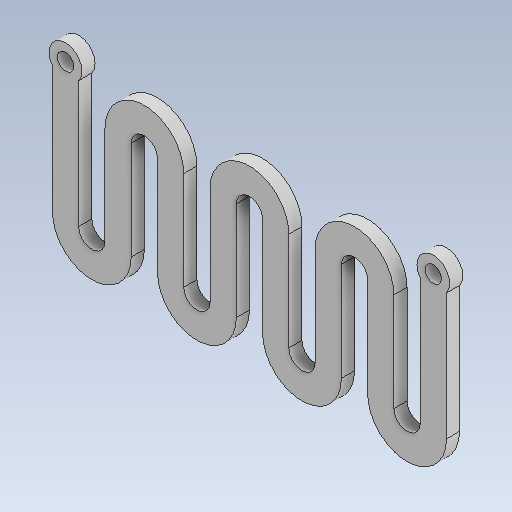
# Autodesk Inventor part: sensor2
Saved by Autodesk Inventor 2025.2 (Build 292293000, 293)
## iProperties
Created: 2025-01-23
Part Number: sensor2
Material: Genérico
Document SubType Name: Modeling
Designer: Gustavo Sousa
Density: 1 g/cm^3
Appearance: Padrão
Author: Gustavo Sousa
Autodesk Inventor part; units mm, degrees
ref_plane "YZ Plane" through (0, 0, 0) normal (1, 0, 0) x (0, 1, 0)
ref_plane "XZ Plane" through (0, 0, 0) normal (0, 1, 0) x (-1, 0, 0)
ref_plane "XY Plane" through (0, 0, 0) normal (0, 0, 1) x (1, 0, 0)
sketch "Esboço1" plane through (0, 0, 0) normal (0, 0, 1) x (1, 0, 0)
  arc A0 (-2600, 1100) -> (-3000, 1100) centre (-2800, 1250) ccw
  line L0 (-2800, 1250) -> (-2800, -825) construction
  line L1 (-3000, -825) -> (-3000, 1100)
  line L2 (-2600, -825) -> (-2600, 1100)
  arc A1 (-2600, -825) -> (-2200, -825) centre (-2400, -825) ccw
  circle A2 centre (-2400, -825) radius 600 construction
  arc A3 (-3000, -825) -> (-1800, -825) centre (-2400, -825) ccw
  line L3 (-2200, -825) -> (-2200, 675)
  line L4 (-1800, -825) -> (-1800, 675)
  arc A4 (-1400, 675) -> (-1800, 675) centre (-1600, 675) ccw
  circle A5 centre (-1600, 675) radius 600 construction
  arc A6 (-1000, 675) -> (-2200, 675) centre (-1600, 675) ccw
  line L5 (-1400, 675) -> (-1400, -825)
  line L6 (-1000, 675) -> (-1000, -825)
  arc A7 (-1000, -825) -> (-600, -825) centre (-800, -825) ccw
  circle A8 centre (-800, -825) radius 600 construction
  arc A9 (-1400, -825) -> (-200, -825) centre (-800, -825) ccw
  line L7 (600, -825) -> (600, 675)
  line L8 (200, -825) -> (200, 675)
  arc A10 (200, 675) -> (-200, 675) centre (0, 675) ccw
  circle A11 centre (0, 675) radius 600 construction
  arc A12 (600, 675) -> (-600, 675) centre (0, 675) ccw
  line L9 (-200, 675) -> (-200, -825)
  line L10 (-600, 675) -> (-600, -825)
  circle A13 centre (800, -825) radius 600 construction
  arc A14 (600, -825) -> (1000, -825) centre (800, -825) ccw
  arc A15 (200, -825) -> (1400, -825) centre (800, -825) ccw
  line L11 (1000, -825) -> (1000, 675)
  line L12 (1400, -825) -> (1400, 675)
  circle A16 centre (1600, 675) radius 200 construction
  arc A17 (1800, 675) -> (1400, 675) centre (1600, 675) ccw
  circle A18 centre (1600, 675) radius 600 construction
  arc A19 (2200, 675) -> (1000, 675) centre (1600, 675) ccw
  line L13 (1800, 675) -> (1800, -825)
  line L14 (2200, 675) -> (2200, -825)
  arc A20 (2200, -825) -> (2600, -825) centre (2400, -825) ccw
  arc A21 (1800, -825) -> (3000, -825) centre (2400, -825) ccw
  arc A22 (3000, 1100) -> (2600, 1100) centre (2800, 1250) ccw
  line L15 (2800, 1250) -> (2800, -825) construction
  line L16 (3000, -825) -> (3000, 1100)
  line L17 (2600, -825) -> (2600, 1100)
  circle A23 centre (-2800, 1250) radius 125
  circle A24 centre (2800, 1250) radius 125
  circle A25 centre (2400, -825) radius 200 construction
  circle A26 centre (2400, -825) radius 600 construction
  point P0 (0, 0)
  point P1 (-600, 675)
  point P2 (-1000, 675)
  dimension "d36" = 1500
  dimension "d46" = 250
  dimension "d47" = 250
  constraints: 38 point on circle, 36 end point, 29 horizontal alignment, 23 vertical, 22 centre point, 18 tangent, 9 coincident, 4 concentric, 4 equal radius, 4 parallel, 2 point on line, 31 other
  measures "d36" distance of L3.start L3.end
  measures "d46" diameter of A23
  measures "d47" diameter of A24
extrude "Extrusão1" add sketch "Esboço1" along normal mid plane 200
